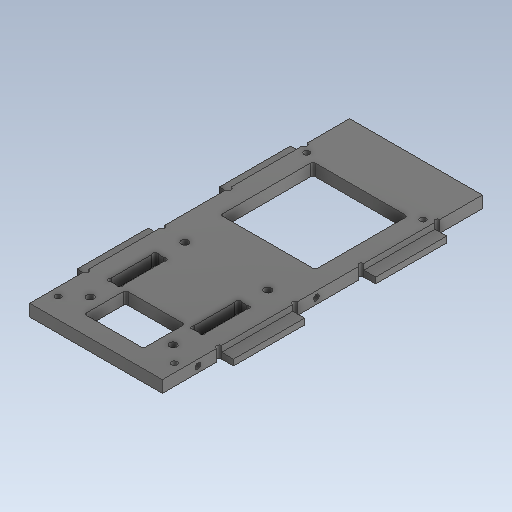
# Autodesk Inventor part: Cockpit_horizontal_frame_02
Saved by Autodesk Inventor 2020 (Build 240168000, 168)
## iProperties
Created: 2021-04-13
Part Number: Cockpit_horizontal_frame_02
Material: アセタール樹脂、黒
Document SubType Name: Modeling
Designer: Masato Kubotera
Density: 1.425 g/cm^3
Appearance: 滑らか - 黒
Mass: 48.5966 g
Surface Area: 179.606 cm^2
Volume: 34.1029 cm^3
d0: 56.000 mm
d1: 130.000 mm
d2: 20.000 mm
d3: 30.000 mm
d4: 30.000 mm
d5: 30.000 mm
d6: 1.050 mm
d7: 1.050 mm
d8: 1.050 mm
d9: 1.050 mm
d10: 5.000 mm
d23: 15.000 mm
d24: 5.000 mm
d25: 20.000 mm
d28: 3.100 mm
d66: 2.500 mm
d67: 0.00 deg
d68: 5.000 mm
d69: 0.00 deg
d72: 75.000 mm
d94: 20.000 mm
d101: 1.000 mm
d103: 8.000 mm
d109: 80.000 mm
Author: Masato Kubotera
Title: Cockpit_horizontal_frame_02
Autodesk Inventor part; units mm, degrees
ref_plane "YZ Plane" through (0, 0, 0) normal (1, 0, 0) x (0, 1, 0)
ref_plane "XZ Plane" through (0, 0, 0) normal (0, 1, 0) x (-1, 0, 0)
ref_plane "XY Plane" through (0, 0, 0) normal (0, 0, 1) x (1, 0, 0)
sketch "スケッチ1" plane through (0, 0, 0) normal (0, 0, 1) x (1, 0, 0)
  line L0 (-28, 65) -> (28, 65)
  line L1 (28, 65) -> (28, 47.1)
  line L2 (-28, -65) -> (-28, -47.1)
  line L3 (-28, 65) -> (28, -65) construction
  line L4 (28, 65) -> (-28, -65) construction
  line L5 (-28, 45) -> (-33, 45)
  line L6 (-33, 15) -> (-28, 15)
  line L7 (-33, 15) -> (-33, 45)
  line L8 (-28, -15) -> (-33, -15)
  line L9 (-33, -15) -> (-33, -45)
  line L10 (-33, -45) -> (-28, -45)
  arc A0 (-28, 45) -> (-28, 47.1) centre (-28, 46.05) ccw
  arc A1 (-28, 12.9) -> (-28, 15) centre (-28, 13.95) ccw
  arc A2 (-28, -15) -> (-28, -12.9) centre (-28, -13.95) ccw
  arc A3 (-28, -47.1) -> (-28, -45) centre (-28, -46.05) ccw
  line L11 (-28, 47.1) -> (-28, 65)
  line L12 (-28, 12.9) -> (-28, 15) construction
  line L13 (-28, -12.9) -> (-28, 12.9)
  line L14 (-28, -47.1) -> (-28, -45) construction
  line L15 (0, 65) -> (0, -65) construction
  arc A4 (28, -45) -> (28, -47.1) centre (28, -46.05) ccw
  line L16 (33, -45) -> (28, -45)
  line L17 (33, -15) -> (33, -45)
  line L18 (28, -15) -> (33, -15)
  arc A5 (28, -12.9) -> (28, -15) centre (28, -13.95) ccw
  arc A6 (28, 15) -> (28, 12.9) centre (28, 13.95) ccw
  line L19 (33, 15) -> (33, 45)
  line L20 (33, 15) -> (28, 15)
  line L21 (28, 45) -> (33, 45)
  arc A7 (28, 47.1) -> (28, 45) centre (28, 46.05) ccw
  line L22 (28, 47.1) -> (28, 45) construction
  line L23 (28, 12.9) -> (28, -12.9)
  line L24 (28, -47.1) -> (28, -65)
  line L25 (28, -12.9) -> (28, -15) construction
  line L26 (-28, -15) -> (-28, -12.9) construction
  line L27 (-28, -45) -> (-28, -15)
  line L28 (28, -15) -> (28, -45)
  line L29 (28, -45) -> (28, -47.1) construction
  line L30 (-20, -25) -> (-15, -25) construction
  line L31 (-15, -25) -> (-15, -45) construction
  line L32 (-15, -45) -> (-20, -45) construction
  line L33 (-20, -45) -> (-20, -25) construction
  line L34 (-20, -25) -> (-15, -45) construction
  line L35 (-15, -25) -> (-20, -45) construction
  line L36 (-20, 2.5) -> (-15, 2.5) construction
  line L37 (-15, 2.5) -> (-15, -72.5) construction
  line L38 (-15, -72.5) -> (-20, -72.5) construction
  line L39 (-20, -72.5) -> (-20, 2.5) construction
  line L40 (-20, 2.5) -> (-15, -72.5) construction
  line L41 (-15, 2.5) -> (-20, -72.5) construction
  circle A8 centre (-17.5, -55) radius 1.55
  line L42 (-20, -35) -> (-15, -35) construction
  line L43 (-17.5, 2.5) -> (-17.5, -72.5) construction
  circle A9 centre (-17.5, -15) radius 1.55
  circle A10 centre (17.5, -55) radius 1.55
  circle A11 centre (17.5, -15) radius 1.55
  line L44 (28, -65) -> (12.5, -65) construction
  line L45 (-12.5, -62.5) -> (-12.5, -45)
  line L46 (-12.5, -45) -> (0, -45)
  line L47 (12.5, -62.5) -> (12.5, -45)
  line L48 (12.5, -45) -> (0, -45)
  line L49 (-12.5, -65) -> (-28, -65) construction
  line L50 (12.5, -65) -> (-12.5, -65) construction
  line L51 (-28, 45) -> (-28, 47.1) construction
  line L52 (-28, 15) -> (-28, 45)
  line L53 (28, 15) -> (28, 12.9) construction
  line L54 (28, 45) -> (28, 15)
  circle A12 centre (-24.5, 43.5) radius 1.25
  line L55 (-28, 0) -> (28, 0) construction
  line L56 (-28, 46.5) -> (28, 46.5) construction
  circle A13 centre (-24.5, -61.5) radius 1.25
  circle A14 centre (24.5, 43.5) radius 1.25
  circle A15 centre (24.5, -61.5) radius 1.25
  circle A16 centre (-17.5, -55) radius 3 construction
  line L57 (-12.5, -62.5) -> (12.5, -62.5)
  line L58 (-20, 41.5) -> (20, 41.5)
  line L59 (20, 2.5) -> (-20, 2.5)
  line L60 (-20, 2.5) -> (-20, 41.5)
  line L61 (20, 2.5) -> (20, 41.5)
  line L62 (-20.05, -43.5651) -> (-18.5651, -45.05) construction
  line L63 (-19.3075, -44.3075) -> (-20.05, -45.05) construction
  arc A17 (-20.05, -43.5651) -> (-18.5651, -45.05) centre (-19.3075, -44.3075) ccw
  line L64 (-20.05, -24.95) -> (-18.5651, -24.95) construction
  line L65 (-14.95, -24.95) -> (-14.95, -26.4349) construction
  line L66 (-14.95, -45.05) -> (-16.4349, -45.05) construction
  line L67 (-20.05, -45.05) -> (-20.05, -43.5651) construction
  line L68 (-20.05, -24.95) -> (-14.95, -45.05) construction
  line L69 (-14.95, -24.95) -> (-20.05, -45.05) construction
  arc A18 (-16.4349, -45.05) -> (-14.95, -43.5651) centre (-15.6925, -44.3075) ccw
  arc A19 (-18.5651, -24.95) -> (-20.05, -26.4349) centre (-19.3075, -25.6925) ccw
  arc A20 (-14.95, -26.4349) -> (-16.4349, -24.95) centre (-15.6925, -25.6925) ccw
  line L70 (-20.05, -43.5651) -> (-20.05, -26.4349)
  line L71 (-18.5651, -45.05) -> (-20.05, -45.05) construction
  line L72 (-16.4349, -45.05) -> (-18.5651, -45.05)
  line L73 (-14.95, -43.5651) -> (-14.95, -45.05) construction
  line L74 (-20.05, -26.4349) -> (-20.05, -24.95) construction
  line L75 (-18.5651, -24.95) -> (-16.4349, -24.95)
  line L76 (-16.4349, -24.95) -> (-14.95, -24.95) construction
  line L77 (-14.95, -26.4349) -> (-14.95, -43.5651)
  arc A21 (18.5651, -45.05) -> (20.05, -43.5651) centre (19.3075, -44.3075) ccw
  arc A22 (14.95, -43.5651) -> (16.4349, -45.05) centre (15.6925, -44.3075) ccw
  arc A23 (16.4349, -24.95) -> (14.95, -26.4349) centre (15.6925, -25.6925) ccw
  arc A24 (20.05, -26.4349) -> (18.5651, -24.95) centre (19.3075, -25.6925) ccw
  line L78 (20.05, -43.5651) -> (20.05, -26.4349)
  line L79 (16.4349, -45.05) -> (18.5651, -45.05)
  line L80 (18.5651, -24.95) -> (16.4349, -24.95)
  line L81 (14.95, -26.4349) -> (14.95, -43.5651)
  line L82 (-28, -65) -> (-28, -70)
  line L83 (-28, -70) -> (28, -70)
  line L84 (28, -70) -> (28, -65)
  point P0 (0, 0)
  point P1 (0, 0)
  point P2 (0, 0)
  point P3 (28, 45)
  point P4 (-17.5, -35)
  point P5 (28, 45)
  dimension "d0" = 56
  dimension "d1" = 130
  dimension "d2" = 20
  dimension "d3" = 30
  dimension "d4" = 30
  dimension "d5" = 30
  dimension "d6" = 1.05
  dimension "d7" = 1.05
  dimension "d8" = 1.05
  dimension "d9" = 1.05
  dimension "d10" = 5
  dimension "d23" = 15
  dimension "d24" = 5
  dimension "d25" = 20
  dimension "d28" = 3.1
  dimension "d72" = 75
  dimension "d94" = 20
  dimension "d103" = 8
  dimension "d109" = 80
  dimension "d111" = 20
  dimension "d113" = 3.5
  dimension "d114" = 2.5
  dimension "d115" = 18.5
  dimension "d116" = 3
  dimension "d117" = 2.5
  dimension "d118" = 3.5
  dimension "d119" = 3.5
  dimension "d120" = 25
  dimension "d121" = 6
  dimension "d124" = 2.5
  dimension "d125" = 7.5
  dimension "d126" = 8
  dimension "d128" = 5
  dimension "d130" = 1.05
  dimension "d131" = 0.05
  dimension "d132" = 0.05
  dimension "d133" = 5
  constraints: 168 end point, 95 parallel, 52 perpendicular, 46 symmetric about line, 40 point on circle, 25 centre point, 22 midpoint, 15 horizontal, 10 vertical, 6 point on line, 3 coincident, 3 collinear, 30 other
  measures "d0" distance of L0.start L0.end
  measures "d1" distance of L0.end L3.end
  measures "d2" distance between parallel lines of L5 L0
  measures "d3" distance of L6.start L5.end
  measures "d4" distance between parallel lines of L8 L6
  measures "d5" distance of L8.end L9.end
  measures "d6" radius of A0
  measures "d7" radius of A1
  measures "d8" radius of A2
  measures "d9" radius of A3
  measures "d10" distance between parallel lines of L7 L11
  measures "d23" distance between parallel lines of L15 L31
  measures "d24" distance of L31.end L32.end
  measures "d25" distance of L30.end L31.end
  measures "d28" diameter of A8
  measures "d72" distance of L36.end L37.end
  measures "d94" distance of A8.centre point (-17.5, -35)
  measures "d109" distance from line of L0 A9.centre
  measures "d111" distance between parallel lines of L44 L46
  measures "d113" distance from line of A12.centre L11
  measures "d114" diameter of A12
  measures "d115" distance between parallel lines of L56 L0
  measures "d116" distance from line of L56 A12.centre
  measures "d117" diameter of A13
  measures "d119" distance from line of L49 A13.centre
  measures "d120" distance between parallel lines of L47 L45
  measures "d121" diameter of A16
  measures "d124" distance between parallel lines of L50 L57
  measures "d125" distance between parallel lines of L49 L38
  measures "d126" distance between parallel lines of L60 L52
  measures "d128" distance between parallel lines of L58 L56
  measures "d130" radius of A17
  measures "d131" distance between parallel lines of L72 L32
  measures "d132" distance between parallel lines of L70 L39
  measures "d133" distance of L4.end L82.end
extrude "押し出し1" add sketch "スケッチ1" along normal blind 2.5
extrude "押し出し2" add sketch "スケッチ1" along normal blind 5 contours L0 L1 A7 L54 A6 L23 A5 L28 A4 L24 L84 L83 L82 L2 A3 L27 A2 L13 A1 L52 A0 L11
fillet "フィレット1" radius 1 7 edges at (-12.5, -45, 2.5) (-12.5, -62.5, 2.5) (12.5, -62.5, 2.5) (-20, 41.5, 2.5) (20, 41.5, 2.5) (20, 2.5, 2.5) (-20, 2.5, 2.5)
sketch "スケッチ7" plane through (28, -70, 0) normal (1, 0, 0) x (0, 0, -1)
  line L0 (0, 55) -> (-2.5, 55) projected
  line L1 (0, 57.1) -> (0, 82.9) projected
  line L2 (0, 0) -> (0, 22.9) projected
  point P0 (0, 70)
  point P1 (-2.5, 15)
  point P2 (-2.5, 65)
  point P3 (0, 25)
  dimension "d136" = 10
  dimension "d137" = 10
  dimension "d138" = 2.5
  dimension "d139" = 2.5
  measures "d136" vertical distance of point (0, 25) point (-2.5, 15)
  measures "d137" distance from line of point (-2.5, 65) L0
  measures "d138" distance from line of L1 point (-2.5, 65)
  measures "d139" distance from line of L2 point (-2.5, 15)
hole "穴6" at (28, -55, 2.5) at (28, -5, 2.5) direction (-1, 0, 0) diameter 2.459 depth 4 thread size "M3x0.5" class "6H" standard "ISO Metric profile"
sketch "スケッチ8" plane through (-28, -70, 0) normal (-1, 0, 0) x (0, 0, 1)
  circle A0 centre (2.5, 15) radius 1.2295 projected
  circle A1 centre (2.5, 65) radius 1.2295 projected
  point P0 (0, 70)
  constraints: 2 coincident
hole "穴7" at (-28, -5, 2.5) at (-28, -55, 2.5) direction (1, 0, 0) diameter 2.459 depth 4 thread size "M3x0.5" class "6H" standard "ISO Metric profile"
equation "\"d2\" = -0.5 * d4 + 0.5 * d1 - d3"
equation "\"d5\" = d3"
equation "\"d7\" = d6"
equation "\"d8\" = d7"
equation "\"d9\" = d8"
